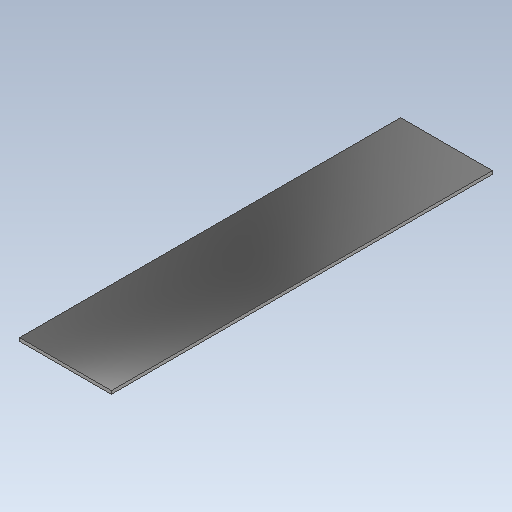
# Autodesk Inventor part: plexiglass1
Saved by Autodesk Inventor 2021 (Build 250183000, 183)
## iProperties
Created: 2021-03-23
Part Number: plexiglass1
Material: Generic
Document SubType Name: Modeling
Designer: con_c_000
Density: 1 g/cm^3
Appearance: Default
Author: con_c_000
Autodesk Inventor part; units mm, degrees
ref_plane "YZ Plane" through (0, 0, 0) normal (1, 0, 0) x (0, 1, 0)
ref_plane "XY Plane" through (0, 0, 0) normal (0, 0, 1) x (1, 0, 0)
ref_plane "Work Plane1" through (0, -280.9875, 0) normal (0, 1, 0) x (-1, 0, 0)
sketch "Sketch1" plane through (0, -280.9875, 0) normal (0, 1, 0) x (-1, 0, 0)
  line L0 (-17.5545, -151.5833) -> (55.8597, -151.5833)
  line L1 (55.8597, -151.5833) -> (55.8597, 153.2167)
  line L2 (55.8597, 153.2167) -> (-17.5545, 153.2167)
  line L3 (-17.5545, 153.2167) -> (-17.5545, -151.5833)
  line L4 (-17.5545, 261.1667) -> (-17.5545, -259.5333)
  line L5 (55.8597, -126.1833) -> (55.8597, -151.5833)
  point P0 (0, 0)
  point P1 (-17.5545, -126.1833)
  point P2 (-17.5545, 127.8167)
  constraints: 12 end point, 2 parallel, 1 horizontal, 1 perpendicular, 5 other
extrude "Extrusion1" add sketch "Sketch1" along normal blind 2.54
body "Solid1"
